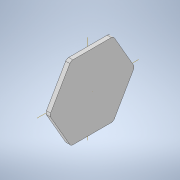
# Autodesk Inventor part: crank case cover
Saved by Autodesk Inventor 2021.1 (Build 251245000, 245)
## iProperties
Created: 2020-08-29
Part Number: crank case cover
Material: Generic
Document SubType Name: Sheet Metal
Designer: Vamshi
Density: 1 g/cm^3
Sheet Metal Rule: Default
Appearance: Default
Author: Vamshi
Autodesk Inventor part; units mm, degrees
ref_plane "YZ Plane" through (0, 0, 0) normal (1, 0, 0) x (0, 1, 0)
ref_plane "XZ Plane" through (0, 0, 0) normal (0, 1, 0) x (-1, 0, 0)
ref_plane "XY Plane" through (0, 0, 0) normal (0, 0, 1) x (1, 0, 0)
sketch "Sketch1" plane through (0, 0, 0) normal (0, 0, 1) x (1, 0, 0)
  line L0 (70.3905, -134.62) -> (-70.3905, -134.62)
  line L1 (-81.3891, -128.27) -> (-151.7796, -6.35)
  line L2 (-151.7796, 6.35) -> (-81.3891, 128.27)
  line L3 (-70.3905, 134.62) -> (70.3905, 134.62)
  line L4 (81.3891, 128.27) -> (151.7796, 6.35)
  line L5 (151.7796, -6.35) -> (81.3891, -128.27)
  arc A0 (-70.3905, 134.62) -> (-81.3891, 128.27) centre (-70.3905, 121.92) ccw
  arc A1 (-151.7796, 6.35) -> (-151.7796, -6.35) centre (-140.7811, 0) ccw
  arc A2 (-81.3891, -128.27) -> (-70.3905, -134.62) centre (-70.3905, -121.92) ccw
  arc A3 (70.3905, -134.62) -> (81.3891, -128.27) centre (70.3905, -121.92) ccw
  arc A4 (151.7796, -6.35) -> (151.7796, 6.35) centre (140.7811, 0) ccw
  arc A5 (81.3891, 128.27) -> (70.3905, 134.62) centre (70.3905, 121.92) ccw
  point P0 (0, 0)
  point P1 (0, 0)
  point P2 (77.7229, -134.62)
  point P3 (-77.7229, -134.62)
  point P4 (-155.4458, 0)
  point P5 (-77.7229, 134.62)
  point P6 (77.7229, 134.62)
  point P7 (155.4458, 0)
  dimension "d0" = 269.24
  dimension "d1" = 12.7
  constraints: 12 end point, 12 point on circle, 12 point on line, 12 tangent, 6 centre point, 5 equal radius, 1 coincident, 1 horizontal, 13 other
  measures "d0" distance between parallel lines of L0 L3
  measures "d1" radius of A0
extrude "Extrusion1" add sketch "Sketch1" along normal blind 15.24
equation "\"BendRadius\" = Thickness"
equation "\"BendReliefWidth\" = Thickness"
equation "\"BendReliefDepth\" = 0.5 * Thickness"
equation "\"CornerReliefSize\" = 4 * Thickness"
equation "\"MinimumRemnant\" = 2 * Thickness"
equation "\"TransitionRadius\" = BendRadius"
equation "\"JacobiRadiusSize\" = BendRadius"
equation "\"GapSize\" = Thickness"
equation "\"Thickness\" = 3.048"
body "Solid1"
